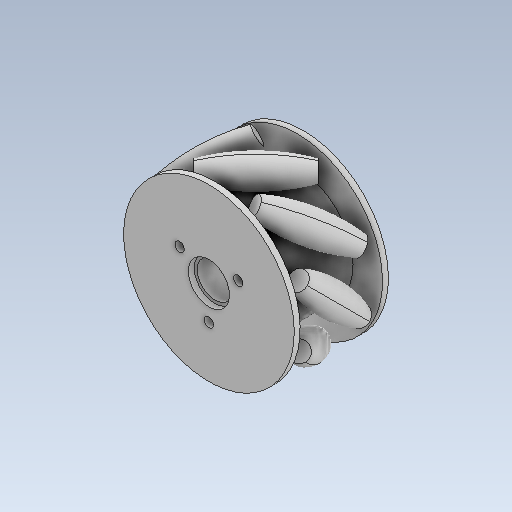
# Autodesk Inventor part: mecanumR
Saved by Autodesk Inventor 2027.1 (Build 311270010, 270A)
## iProperties
Created: 2026-10-09
Part Number: mecanumR
Material: 一般
Document SubType Name: Modeling
Designer: ug_nd
Density: 1 g/cm^3
Appearance: 既定
Author: ug_nd
Autodesk Inventor part; units mm, degrees
ref_plane "XZ Plane" through (0, 0, 0) normal (0, 1, 0) x (-1, 0, 0)
ref_plane "XY Plane" through (0, 0, 0) normal (0, 0, 1) x (1, 0, 0)
sketch "スケッチ1" plane through (0, 0, 0) normal (0, 0, 1) x (1, 0, 0)
  circle A0 centre (0, 0) radius 30
  circle A1 centre (0, 0) radius 6
  dimension "d0" = 12
  dimension "d1" = 60
  constraints: 2 centre point, 2 coincident
  measures "d0" diameter of A1
  measures "d1" diameter of A0
extrude "押し出し1" add sketch "スケッチ1" along normal mid plane 32
sketch "スケッチ3" plane through (0, 0, 16) normal (0, 0, 1) x (1, 0, 0)
  circle A0 centre (0, 0) radius 11.5 construction
  circle A1 centre (-9.9593, 5.75) radius 1.6
  circle A2 centre (0, -11.5) radius 1.6
  circle A3 centre (9.9593, 5.75) radius 1.6
  dimension "d7" = 23
  dimension "d8" = 3.2
  dimension "d11" = 360
  constraints: 3 centre point, 1 coincident, 1 vertical alignment, 10 other
  measures "d8" diameter of A1
extrude "押し出し3" cut sketch "スケッチ3" against normal through all
sketch "スケッチ2" plane through (0, 0, 16) normal (0, 0, 1) x (1, 0, 0)
  circle A0 centre (0, 0) radius 7
  dimension "d4" = 14
  constraints: 1 centre point, 1 coincident
  measures "d4" diameter of A0
extrude "押し出し2" cut sketch "スケッチ2" against normal blind 2
mirror "ミラー1" about plane through (0, 0, 0) normal (0, 0, 1) of "押し出し2"
ref_plane "作業平面1" through (0, 0, 0) normal (0.7071068, 0, -0.7071068) x (0, 1, 0)
sketch "スケッチ4" plane through (0, 0, 0) normal (0.7071068, 0, -0.7071068) x (0, 1, 0)
  ellipse E0 centre (-11.5, 0) end of major axis (-11.5, 2.2627) minor radius 1.6 construction
  ellipse E1 centre (5.75, 14.0846) end of major axis (5.75, 16.3473) minor radius 1.6 construction
  ellipse E2 centre (5.75, -14.0846) end of major axis (5.75, -11.8218) minor radius 1.6 construction
  ellipse E3 centre (0, 0) end of major axis (0, -8.4853) minor radius 6 construction
  line L0 (25, -23.4521) -> (25, 23.4521) construction
  line L1 (-42, 0) -> (42, 0) construction
  line L2 (0, -50.0996) -> (0, 50.0996) construction
  line L3 (28.0624, -15) -> (25, -15)
  line L4 (28.0624, 15) -> (25, 15)
  line L5 (25, -15) -> (25, 15)
  line L6 (25.3772, -22.6274) -> (-25.3772, -22.6274) projected
  ellipse E4 centre (0, 0) end of major axis (0, 42.4264) minor radius 30 (-25.3772, 22.6274) -> (-25.3772, -22.6274) ccw projected
  line L7 (-25.3772, 22.6274) -> (25.3772, 22.6274) projected
  ellipse E5 centre (0, 0) end of major axis (0, 42.4264) minor radius 30 (25.3772, -22.6274) -> (25.3772, 22.6274) ccw projected
  point P0 (25, 0)
  dimension "d16" = 50
  dimension "d17" = 30
  constraints: 8 end point, 2 point on line, 2 symmetric about line, 1 horizontal, 1 midpoint, 1 vertical, 6 other
  measures "d16" diameter of L0 L2
  measures "d17" distance between parallel lines of L4 L3
sketch "スケッチ5" plane through (0, 0, 0) normal (1, 0, 0) x (0, 1, 0)
  line L0 (7, 14) -> (7, 16) construction
  line L1 (7, 16) -> (30, 16) projected
  line L2 (30, 16) -> (30, -16) projected
  line L3 (30, -16) -> (7, -16) projected
  line L4 (7, -16) -> (7, -14) construction
  line L5 (7, -14) -> (6, -14) construction
  line L6 (6, -14) -> (6, 14) construction
  line L7 (6, 14) -> (7, 14) construction
  line L8 (-13.1, 16) -> (-13.1, -16) construction
  line L9 (-13.1, -16) -> (-30, -16) construction
  line L10 (-30, -16) -> (-30, 16) construction
  line L11 (-30, 16) -> (-13.1, 16) construction
  line L12 (-9.9, -16) -> (-9.9, 16) construction
  line L13 (-9.9, 16) -> (-7, 16) construction
  line L14 (-7, 16) -> (-7, 14) construction
  line L15 (-7, 14) -> (-6, 14) construction
  line L16 (-6, 14) -> (-6, -14) construction
  line L17 (-6, -14) -> (-7, -14) construction
  line L18 (-7, -14) -> (-7, -16) construction
  line L19 (-7, -16) -> (-9.9, -16) construction
  line L20 (29, 16) -> (29, 14)
  line L21 (-42, 0) -> (42, 0) construction
  line L22 (29, 14) -> (19, 14)
  line L23 (29, -16) -> (29, -14)
  line L24 (29, -14) -> (19, -14)
  line L25 (19, 14) -> (19, -14)
  line L26 (0, -22.4) -> (0, 22.4) construction
  point P0 (0, 0)
  dimension "d22" = 38
  dimension "d23" = 58
  dimension "d24" = 28
  constraints: 10 end point, 3 symmetric about line, 2 vertical, 1 horizontal, 1 point on line
  measures "d22" diameter of L25 L26
  measures "d23" diameter of L23 L26
  measures "d24" distance between parallel lines of L22 L24
revolve "回転2" cut sketch "スケッチ5" angle 360 about axis through (0, 0, -10) along (0, 0, 1)
revolve "回転1" add sketch "スケッチ4" angle 360 about axis through (-16.5831, 25, -16.5831) along (0.7071068, 0, 0.7071068) contours L3 L5 L4 E5
pattern_circular "円形状パターン1" count 8 over 360 about axis through (0, 0, -10) along (0, 0, 1) of "回転1"
mirror "ミラー2" about plane through (0, 0, 0) normal (1, 0, 0) remove original yes
